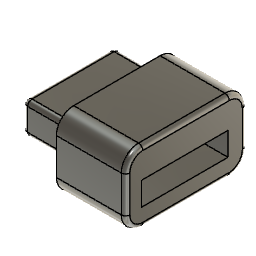
ATS_Plug_PoweredUp_PCB_16mm (Autodesk Fusion 360 design; units mm, degrees)
Autodesk Fusion 360 part; units mm, degrees
sketch "Schizzo1" plane through (0, 0, 0) normal (1, 0, 0) x (0, 1, 0)
  line L0 (0, 0) -> (1.1976, -0.5058)
  line L1 (0, 0) -> (1.3, 0) construction
  line L2 (0, 0) -> (1.816, 4.3)
  line L3 (15, 0) -> (15, 4.3)
  line L4 (1.816, 4.3) -> (15, 4.3)
  line L5 (15, 0) -> (13.7, 0)
  line L6 (1.3, 0) -> (1.3, 2.4)
  line L7 (13.7, 0) -> (13.7, 2.4)
  line L8 (1.3, 2.4) -> (13.7, 2.4)
  constraint horizontal L1
  constraint coincident L0.start L1.start
  constraint perpendicular L0 L2
  constraint vertical L3
  constraint perpendicular L3 L4
  constraint perpendicular L3 L5
  constraint perpendicular L1 L6
  constraint perpendicular L5 L7
  constraint perpendicular L7 L8
sketch "Schizzo2" plane through (0, 0, 0) normal (1, 0, 0) x (0, 1, 0)
sketch "Schizzo3" plane through (0, 0, 0) normal (1, 0, 0) x (0, 1, 0)
  line L0 (0, 0) -> (1, 0)
  line L1 (0, 0) -> (0, 4.3)
  line L2 (0, 4.3) -> (10.5, 4.3)
  line L3 (10.5, 4.3) -> (10.5, 0.7)
  line L4 (10.5, 0.7) -> (9.5, 0.7)
  line L5 (1, 0) -> (1, 2.7)
  line L6 (9.5, 0.7) -> (9.5, 2.7)
  line L7 (1, 2.7) -> (9.5, 2.7)
  constraint coincident L0.start L1.start
  constraint horizontal L0
  constraint perpendicular L0 L1
  constraint horizontal L2
  constraint perpendicular L2 L3
  constraint perpendicular L3 L4
  constraint vertical L5
  constraint perpendicular L4 L6
  constraint perpendicular L6 L7
extrude "Estrudi2" add sketch "Schizzo3" along normal blind 5.5 makes body 1
sketch "Schizzo4" plane through (0, 0, 0) normal (1, 0, 0) x (0, 1, 0)
  line L0 (-15.8951, 4.7827) -> (-1.8951, 4.7827)
  line L1 (-1.8951, 4.7827) -> (-1.8951, -3.2173)
  line L2 (-1.8951, -3.2173) -> (-15.8951, -3.2173)
  line L3 (-15.8951, -3.2173) -> (-15.8951, 4.7827)
  line L4 (-13.0135, 1.5781) -> (-5.0135, 1.5781)
  line L5 (-5.0135, 1.5781) -> (-5.0135, -0.2219)
  line L6 (-5.0135, -0.2219) -> (-13.0135, -0.2219)
  line L7 (-13.0135, -0.2219) -> (-13.0135, 1.5781)
  constraint horizontal L0
  constraint vertical L1
  constraint horizontal L2
  constraint vertical L3
  constraint horizontal L4
  constraint vertical L5
  constraint horizontal L6
  constraint vertical L7
extrude "Estrudi3" add sketch "Schizzo4" along normal blind 8 separate body makes body 2
move_body "Sposta1" bodies 2 to x (1, 0, 0) y (0, 1, 0) z (0, 0, 1) at (6.542, 13.4224, 1.0871)
move_body "Sposta2" bodies 2 to x (1, 0, 0) y (0, 1, 0) z (0, 0, 1) at (-0.1, 0.85, 0.1)
move_face "Sposta faccia1" by (-1, 0, 0) 1 faces at (9.1087, 3.044, 5.9697) on bodies 2
move_body "Sposta3" bodies 2 to x (1, 0, 0) y (0, 1, 0) z (0, 0, 1) at (-1, 0, 0)
fillet "Raccordo1" radius 2 1 edges at (9.442, -1.6226, 5.9697) on bodies 2
fillet "Raccordo2" radius 2 1 edges at (9.442, -1.6226, -2.0303) on bodies 2
fillet "Raccordo3" radius 2 1 edges at (9.442, 12.3774, 5.9697) on bodies 2
fillet "Raccordo4" radius 2 1 edges at (9.442, 12.3774, -2.0303) on bodies 2
fillet "Raccordo5" radius 0.5 1 edges at (0, 10.5, 2.5) on bodies 1
fillet "Raccordo6" radius 0.5 3 edges at (0, 5, 4.3) (0.1464, 10.3536, 4.3) (3, 10.5, 4.3) on bodies 1
fillet "Raccordo7" radius 0.5 3 edges at (0, 0, 1.9) (0.1464, 0, 4.1536) (3, 0, 4.3) on bodies 1
move_face "FacceDiOffset1" offset -0.7 1 faces at (2, 0.6667, 0) on bodies 1
fillet "Raccordo8" radius 0.5 3 edges at (0, 9.75, 0.7) (0.1464, 10.3536, 0.7) (3, 10.5, 0.7) on bodies 1
fillet "Raccordo9" radius 0.5 3 edges at (0, 0.75, 0.7) (0.1464, 0.1464, 0.7) (3, 0, 0.7) on bodies 1
fillet "Raccordo10" radius 0.5 8 edges at (13.442, 11.7916, -1.4445) (13.442, 12.3774, 1.9697) (13.442, 11.7916, 5.3839) (13.442, 5.3774, 5.9697) (13.442, -1.0369, 5.3839) (13.442, -1.6226, 1.9697) (13.442, -1.0369, -1.4445) (13.442, 5.3774, -2.0303) on bodies 2
sketch "Schizzo5" plane through (13.442, 0, 0) normal (1, 0, 0) x (0, 1, 0)
  line L0 (9.259, 0.9651) -> (1.259, 0.9651)
  line L1 (1.259, 0.9651) -> (1.259, 2.7651)
  line L2 (1.259, 2.7651) -> (9.259, 2.7651)
  line L3 (9.259, 2.7651) -> (9.259, 0.9651)
  arc A0 (10.3774, -1.5303) -> (11.8774, -0.0303) centre (10.3774, -0.0303) ccw
  line L4 (11.8774, -0.0303) -> (11.8774, 3.9697)
  arc A1 (11.8774, 3.9697) -> (10.3774, 5.4697) centre (10.3774, 3.9697) ccw
  line L5 (10.3774, 5.4697) -> (0.3774, 5.4697)
  arc A2 (0.3774, 5.4697) -> (-1.1226, 3.9697) centre (0.3774, 3.9697) ccw
  line L6 (-1.1226, 3.9697) -> (-1.1226, -0.0303)
  arc A3 (-1.1226, -0.0303) -> (0.3774, -1.5303) centre (0.3774, -0.0303) ccw
  line L7 (0.3774, -1.5303) -> (10.3774, -1.5303)
  line L8 (-12.5, 4) -> (-2.5, 4)
  line L9 (-2.5, 4) -> (-2.5, 1.8)
  line L10 (-2.5, 1.8) -> (-12.5, 1.8)
  line L11 (-12.5, 1.8) -> (-12.5, 4)
  dimension "d51" = 10
  dimension "d52" = 2.2
  constraint horizontal L8
  constraint vertical L9
  constraint horizontal L10
  constraint vertical L11
  measures "d51" distance of L8.start L8.end
  measures "d52" distance of L8.start L10.end
extrude "Estrudi4" add sketch "Schizzo5" along normal blind 3 separate body contours L8 L9 L10 L11 makes body 3
move_body "Sposta4" bodies 3 to x (1, 0, 0) y (0, 1, 0) z (0, 0, 1) at (0, 13.0325, -1.9868)
move_body "Sposta5" bodies 3 to x (1, 0, 0) y (0, 1, 0) z (0, 0, 1) at (-3, -0.3, 0.3)
move_face "Sposta faccia2" by (0, 0, 5) 1 faces at (13.442, 3.5659, 1.5799) on bodies 3
move_body "Sposta6" bodies 3 to x (1, 0, 0) y (0, 1, 0) z (0, 0, 1) at (0, 0, 0.45)
combine "Unisci1" operation cut target body 2 tool bodies 3
move_face "FacceDiOffset2" offset 0.2 1 faces at (7.942, 3.7107, 5.9697) on bodies 2
move_face "FacceDiOffset3" offset -0.5 1 faces at (11.442, 6.8992, 0.5632) on bodies 2
